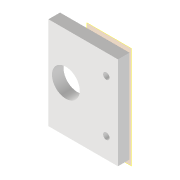
# Autodesk Inventor part: 40_XYZstage_micrometer_motorized_nema8_lightsheet_samplemount_ontop_2
Saved by Autodesk Inventor 2022 (Build 260153000, 153)
## iProperties
Created: 2023-07-30
Part Number: 40_XYZstage_micrometer_motorized_nema8_lightsheet_samplemount_ontop_2
Material: Generisch
Document SubType Name: Modeling
Designer: diederichbenedict
Density: 1 g/cm^3
Appearance: Vorgabe
Author: diederichbenedict
Autodesk Inventor part; units mm, degrees
ref_plane "YZ Plane" through (0, 0, 0) normal (1, 0, 0) x (0, 1, 0)
ref_plane "XZ Plane" through (0, 0, 0) normal (0, 1, 0) x (-1, 0, 0)
ref_plane "XY Plane" through (0, 0, 0) normal (0, 0, 1) x (1, 0, 0)
ref_plane "Arbeitsebene1" through (0, 0, 0) normal (0, 0, 1) x (1, 0, 0)
sketch "Skizze1" plane through (0, 0, 0) normal (0, 0, 1) x (1, 0, 0)
  circle A0 centre (0, 11.25) radius 1.4 projected
  circle A1 centre (0, -11.25) radius 1.4 projected
  line L0 (2.5, 20) -> (-2.5, 20) projected
  line L1 (-2.5, 20) -> (-2.5, 2.5) projected
  line L2 (-10.5, 2.5) -> (-2.5, 2.5) projected
  line L3 (-10.5, -2.5) -> (-10.5, 2.5) projected
  line L4 (-2.5, -2.5) -> (-10.5, -2.5) projected
  line L5 (-2.5, -2.5) -> (-2.5, -20) projected
  line L6 (-2.5, -20) -> (2.5, -20) projected
  line L7 (2.5, -20) -> (2.5, -2.5) projected
  line L8 (5, -2.5) -> (2.5, -2.5) projected
  line L9 (5, 2.5) -> (5, -2.5) projected
  line L10 (2.5, 2.5) -> (5, 2.5) projected
  line L11 (2.5, 2.5) -> (2.5, 20) projected
  line L12 (5, 20) -> (-25, 20)
  line L13 (-25, 20) -> (-25, -20)
  line L14 (-25, -20) -> (5, -20)
  line L15 (5, -20) -> (5, 20)
  circle A2 centre (32.5, 0) radius 1.7096 projected
  circle A3 centre (-17.5, 0) radius 6
  point P0 (0, 0)
  point P1 (5, 0)
  dimension "d0" = 30
  dimension "d1" = 12
  dimension "d2" = 50
  constraints: 8 end point, 2 midpoint, 2 parallel, 1 centre point, 1 horizontal, 1 perpendicular
  measures "d0" distance of L14.end L13.end
  measures "d1" diameter of A3
  measures "d2" distance of A3.centre A2.centre
extrude "Extrusion1" add sketch "Skizze1" along normal blind 5 contours L11 L10 L9 L8 L7 L6 L5 L4 L3 L2 L1 L0 | L12 L15 L10 L11 | L1 L2 L3 L4 L5 L14 L13 L12 | L15 L14 L7 L8
